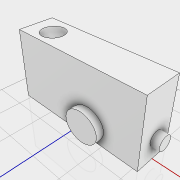
# Autodesk Inventor part: ЛЦМК0000002.00.00.00.00.05
Saved by Autodesk Inventor 2021.2 (Build 252289000, 289)
## iProperties
Created: 2025-10-23
Part Number: ЛЦМК0000002.00.00.00.00.05
Material: Типовые
Document SubType Name: Modeling
Designer: Захаров
Density: 1 g/cm^3
Appearance: Гладкий - белый
Author: Захаров
Autodesk Inventor part; units mm, degrees
ref_plane "YZ Plane" through (0, 0, 0) normal (1, 0, 0) x (0, 1, 0)
ref_plane "XZ Plane" through (0, 0, 0) normal (0, 1, 0) x (-1, 0, 0)
ref_plane "XY Plane" through (0, 0, 0) normal (0, 0, 1) x (1, 0, 0)
sketch "Эскиз1" plane through (0, 0, 0) normal (0, 0, 1) x (1, 0, 0)
  line L0 (-42.8, 22.15) -> (42.8, 22.15)
  line L1 (42.8, 22.15) -> (42.8, -22.15)
  line L2 (42.8, -22.15) -> (-42.8, -22.15)
  line L3 (-42.8, -22.15) -> (-42.8, 22.15)
  line L4 (-42.8, 22.15) -> (42.8, -22.15) construction
  line L5 (42.8, 22.15) -> (-42.8, -22.15) construction
  point P0 (0, 0)
  dimension "d0" = 85.6
  dimension "d1" = 44.3
  constraints: 12 end point, 2 midpoint, 2 parallel, 1 horizontal, 1 perpendicular
  measures "d0" distance of L1.end L2.end
  measures "d1" distance of L0.end L1.end
extrude "Выдавливание1" add sketch "Эскиз1" along normal mid plane 23
sketch "Эскиз2" plane through (0, 0, 11.5) normal (0, 0, 1) x (1, 0, 0)
  line L0 (-1.2, -2.15) -> (20.8, -2.15)
  line L1 (20.8, -2.15) -> (20.8, -22.15)
  line L2 (20.8, -22.15) -> (-1.2, -22.15)
  line L3 (-1.2, -22.15) -> (-1.2, -2.15)
  line L4 (-42.8, -22.15) -> (42.8, -22.15) projected
  line L5 (42.8, -22.15) -> (42.8, 22.15) projected
  ellipse E0 centre (9.8, -12.15) end of major axis (20.8, -12.15) minor radius 10
  point P0 (0, 0)
  point P1 (20.8, -12.15)
  point P2 (9.8, -2.15)
  point P3 (9.8, -22.15)
  point P4 (-1.2, -12.15)
  dimension "d4" = 20
  dimension "d5" = 44
  dimension "d6" = 22
  constraints: 8 end point, 4 midpoint, 2 parallel, 1 horizontal, 1 perpendicular, 1 point on line, 6 other
  measures "d4" distance between parallel lines of L4 L0
  measures "d5" distance between parallel lines of L5 L3
  measures "d6" distance of L1.end L2.end
extrude "Выдавливание2" add sketch "Эскиз2" along normal blind 5 contours E0
sketch "Эскиз3" plane through (42.8, -22.15, 11.5) normal (1, 0, 0) x (0, 0, -1)
  circle A0 centre (12, 13.5) radius 4.5
  line L0 (23, 0) -> (0, 0) projected
  line L1 (0, 0) -> (0, 44.3) projected
  point P0 (11.5, 22.15)
  dimension "d9" = 13.5
  dimension "d10" = 9
  dimension "d22" = 12
  constraints: 1 centre point
  measures "d9" distance from line of L0 A0.centre
  measures "d10" diameter of A0
  measures "d22" distance from line of L1 A0.centre
extrude "Выдавливание3" add sketch "Эскиз3" along normal blind 5
sketch "Эскиз4" plane through (-42.8, -22.15, -11.5) normal (0, -1, 0) x (1, 0, 0)
  circle A0 centre (15.5, 12) radius 7.5
  line L0 (0, 23) -> (0, 0) projected
  line L1 (0, 23) -> (52.6, 23) projected
  point P0 (42.8, 11.5)
  point P1 (41.6, 23)
  dimension "d13" = 15
  dimension "d14" = 15.5
  dimension "d21" = 11
  constraints: 1 centre point
  measures "d13" diameter of A0
  measures "d14" distance from line of L0 A0.centre
  measures "d21" distance from line of L1 A0.centre
extrude "Выдавливание4" cut sketch "Эскиз4" against normal through all
sketch "Эскиз5" plane through (0, 0, -11.5) normal (0, 0, -1) x (-1, 0, 0)
  line L0 (-42.8, -22.15) -> (42.8, -22.15) projected
  line L1 (42.8, -22.15) -> (42.8, 22.15) projected
  line L2 (42.8, 22.15) -> (-42.8, 22.15) projected
  line L3 (-42.8, 22.15) -> (-42.8, -22.15) projected
  line L4 (-40.8, 20.15) -> (40.8, 20.15)
  line L5 (40.8, 20.15) -> (40.8, -20.15)
  line L6 (40.8, -20.15) -> (-40.8, -20.15)
  line L7 (-40.8, -20.15) -> (-40.8, 20.15)
  line L8 (17.8, 20.15) -> (17.8, -20.15)
  dimension "d23" = 2
  dimension "d24" = 23
  constraints: 10 end point, 2 point on line, 1 perpendicular, 3 other
  measures "d23" distance between parallel lines of L2 L4
  measures "d24" distance between parallel lines of L5 L8
extrude "Выдавливание5" cut sketch "Эскиз5" against normal blind 3 contours L4 L5 L6 L8
